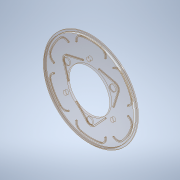
# Autodesk Inventor part: Top Lid
Saved by Autodesk Inventor 2020 (Build 240168000, 168)
## iProperties
Created: 2020-03-28
Part Number: Top Lid
Material: Generic
Document SubType Name: Modeling
Designer: pengpeng
Density: 1 g/cm^3
Appearance: Polycarbonate - Smoked
Author: pengpeng
Autodesk Inventor part; units mm, degrees
ref_plane "YZ Plane" through (0, 0, 0) normal (1, 0, 0) x (0, 1, 0)
ref_plane "XY Plane" through (0, 0, 0) normal (0, 0, 1) x (1, 0, 0)
sketch "Sketch1" plane through (0, 0, 0) normal (0, 0, 1) x (1, 0, 0)
  circle A0 centre (0, 0) radius 68
  dimension "d1" = 136
  constraints: 1 centre point
  measures "d1" diameter of A0
extrude "Extrusion1" add sketch "Sketch1" along normal blind 80
shell "Shell1" thickness 3 removed faces 1 at (13.6377, 7.7647, 0)
sketch "Sketch2" plane through (0, 0, 80) normal (0, 0, 1) x (1, 0, 0)
  circle A0 centre (0, 0) radius 32
  dimension "d5" = 64
  constraints: 1 centre point, 1 coincident
  measures "d5" diameter of A0
extrude "Extrusion2" cut sketch "Sketch2" against normal up to surface (3 mm away)
sketch "Sketch3" plane through (0, 0, 77) normal (0, 0, -1) x (-1, 0, 0)
  circle A0 centre (0, 0) radius 32 projected
  circle A1 centre (0, 0) radius 65 projected
  circle A2 centre (0, -40) radius 4.8
  line L0 (0, 0) -> (0, -56.282) construction
  line L1 (0, 0) -> (-47.9956, 27.7103) construction
  line L2 (0, 0) -> (60.1339, 34.7183) construction
  circle A3 centre (-34.641, 20) radius 4.8
  circle A4 centre (34.641, 20) radius 4.8
  dimension "d8" = 9.6
  dimension "d9" = 40
  dimension "d10" = 120
  dimension "d11" = 120
  dimension "d12" = 9.6
  dimension "d13" = 9.6
  dimension "d14" = 40
  dimension "d15" = 40
  constraints: 6 end point, 3 centre point, 2 point on line, 1 vertical
  measures "d8" diameter of A2
  measures "d9" distance of point (0, 0) A2.centre
  measures "d10" angle of L0 L1
  measures "d11" angle of L0 L2
  measures "d12" diameter of A3
  measures "d13" diameter of A4
  measures "d14" distance of point (0, 0) A4.centre
  measures "d15" distance of point (0, 0) A3.centre
extrude "Extrusion3" cut sketch "Sketch3" against normal blind 1.524 contours A2 | A3 | A4
ref_plane "Work Plane1" through (0, 0, 55) normal (0, 0, 1) x (1, 0, 0)
sketch "Sketch4" plane through (0, 0, 55) normal (0, 0, 1) x (1, 0, 0)
  circle A0 centre (0, 0) radius 68 projected
  circle A1 centre (0, 0) radius 68 projected
  line L0 (0, 68) -> (56.3915, 68)
  line L1 (56.3915, 68) -> (56.3915, 38)
  line L2 (56.3915, 38) -> (0, 38)
  line L3 (0, 38) -> (0, 68)
  dimension "d24" = 30
  constraints: 8 end point, 2 horizontal, 2 parallel, 1 perpendicular, 1 vertical alignment, 3 other
  measures "d24" distance between parallel lines of L2 L0
extrude "Extrusion4" add sketch "Sketch4" against normal blind 25 contours A0 L0 L1
sketch "Sketch6" plane through (56.3915, 38, 55) normal (1, 0, 0) x (0, 0, -1)
  line L0 (0, 0) -> (0, 30) projected
  line L1 (25, 0) -> (0, 0) projected
  line L2 (25, 30) -> (25, 0) projected
  line L3 (0, 30) -> (25, 30) projected
  line L4 (22, 27) -> (22, 3)
  line L5 (22, 3) -> (3, 3)
  line L6 (3, 3) -> (3, 27)
  line L7 (3, 27) -> (22, 27)
  point P0 (55, -38)
  dimension "d27" = 3
  constraints: 8 end point, 3 other
  measures "d27" distance between parallel lines of L3 L7
extrude "Extrusion5" cut sketch "Sketch6" against normal blind 56.391 contours L4 L5 L6 L7
ref_plane "Work Plane4" through (0, 68, 0) normal (0, 1, 0) x (-1, 0, 0)
sketch "Sketch9" plane through (56.3915, 38, 55) normal (1, 0, 0) x (0, 0, -1)
  line L0 (3, 3) -> (3, 27) projected
  line L1 (3, 27) -> (22, 27) projected
  line L2 (22, 27) -> (22, 3) projected
  line L3 (22, 3) -> (3, 3) projected
  line L4 (0, 0) -> (0, 30) projected
  line L5 (25, 0) -> (0, 0) projected
  line L6 (25, 30) -> (25, 0) projected
  line L7 (0, 30) -> (25, 30) projected
  point P0 (55, -38)
sketch "Sketch10" plane through (0, 68, 0) normal (0, 1, 0) x (-1, 0, 0)
  circle A0 centre (-56.3915, 0) radius 55 construction
  line L0 (-127.7058, 55) -> (100.6176, 55) projected
  line L1 (-56.3915, 55) -> (0, 55) projected
  line L2 (0, 0) -> (-96.3915, 0) construction
  arc A1 (-56.3915, 55) -> (-111.3915, 0) centre (-56.3915, 0) ccw
  constraints: 4 point on circle, 2 centre point, 2 coincident, 2 end point, 1 horizontal, 1 point on line, 1 tangent
sweep "Sweep2" add profiles "Sketch9" path "Sketch10" path curves A1
sketch "Sketch11" plane through (0, 0, 77) normal (0, 0, -1) x (-1, 0, 0)
  circle A0 centre (-34.641, 20) radius 4.8 projected
  circle A1 centre (34.641, 20) radius 4.8 projected
  circle A2 centre (0, -40) radius 4.8 projected
  circle A3 centre (0, 0) radius 32 projected
  circle A4 centre (0, 0) radius 65 projected
  circle A5 centre (-34.641, 20) radius 6.3
  circle A6 centre (34.641, 20) radius 6.3
  circle A7 centre (0, -40) radius 6.3
  circle A8 centre (0, 0) radius 33.5
  line L0 (-36.0415, 26.1424) -> (-7.4468, 32.6618)
  line L1 (-40.6607, 18.1416) -> (-32.0094, -9.8818)
  line L2 (36.0415, 26.1424) -> (7.4468, 32.6618)
  line L3 (40.6607, 18.1416) -> (32.0094, -9.8818)
  line L4 (4.6192, -44.284) -> (24.5626, -22.78)
  line L5 (-4.6192, -44.284) -> (-24.5626, -22.78)
  circle A9 centre (-34.641, 20) radius 7.8
  line L6 (-42.0939, 17.6992) -> (-34.7194, -6.1884)
  circle A10 centre (34.641, 20) radius 7.8
  circle A11 centre (0, -40) radius 7.8
  line L7 (-36.3749, 27.6048) -> (-12.0004, 33.1621)
  line L8 (36.3749, 27.6048) -> (12.0004, 33.1621)
  line L9 (42.0939, 17.6992) -> (34.7194, -6.1884)
  line L10 (5.7191, -45.304) -> (22.7191, -26.9737)
  line L11 (-5.7191, -45.304) -> (-22.7191, -26.9737)
  line L12 (-34.7194, -6.1884) -> (-33.2862, -5.746)
  line L13 (-22.7191, -26.9737) -> (-21.6192, -25.9537)
  line L14 (12.0004, 33.1621) -> (11.6669, 31.6997)
  line L15 (34.7194, -6.1884) -> (33.2862, -5.746)
  line L16 (22.7191, -26.9737) -> (21.6192, -25.9537)
  line L17 (-12.0004, 33.1621) -> (-11.6669, 31.6997)
  dimension "d39" = 1.5
  dimension "d40" = 1.5
  dimension "d41" = 1.5
  dimension "d42" = 1.5
  dimension "d43" = 1.5
  dimension "d44" = 1.5
  dimension "d45" = 1.5
  dimension "d46" = 25
  dimension "d47" = 25
  dimension "d48" = 25
  dimension "d49" = 25
  dimension "d50" = 25
  dimension "d51" = 25
  constraints: 36 end point, 18 point on circle, 18 tangent, 7 centre point, 6 parallel, 6 perpendicular, 6 point on line
  measures "d39" radial gap between concentric circles of A0 A5
  measures "d40" radial gap between concentric circles of A1 A6
  measures "d41" radial gap between concentric circles of A2 A7
  measures "d42" radial gap between concentric circles of A8 A3
  measures "d43" radial gap between concentric circles of A5 A9
  measures "d44" radial gap between concentric circles of A6 A10
  measures "d45" radial gap between concentric circles of A7 A11
  measures "d46" distance of L6.start L6.end
  measures "d47" distance of L7.start L7.end
  measures "d48" distance of L8.start L8.end
  measures "d49" distance of L9.start L9.end
  measures "d50" distance of L10.start L10.end
  measures "d51" distance of L11.start L11.end
extrude "Extrusion6" add sketch "Sketch11" along normal blind 1.5 contours A5 L1 A9 L0 | A9 L7 L17 L0 | L1 L12 L6 A9 | L14 L8 A10 L2 | L5 A11 L11 L13 | A10 L3 A6 L2 | L5 A7 L4 A11 | A10 L9 L15 L3 | L16 L10 A11 L4
sketch "Sketch14" plane through (0, 0, 80) normal (0, 0, 1) x (1, 0, 0)
  circle A0 centre (0, 0) radius 32 projected
  line L0 (0, 0) -> (0, 28.9416) construction
  circle A1 centre (0, 41) radius 3
  line L1 (0, 0) -> (-25.0642, -14.4708) construction
  line L2 (0, 0) -> (25.0642, -14.4708) construction
  point P0 (-35.507, -20.5)
  point P1 (-35.507, -20.5)
  point P2 (35.507, -20.5)
  point P3 (35.507, -20.5)
  dimension "d98" = 6
  dimension "d99" = 41
  dimension "d102" = 360
  constraints: 6 end point, 3 coincident, 3 point on line, 1 centre point, 1 vertical, 16 other
  measures "d98" diameter of A1
  measures "d99" distance of point (0, 0) A1.centre
hole "Hole1" at (0, 41, 80) at (-35.507, -20.5, 80) at (35.507, -20.5, 80) direction (0, 0, -1) diameter 6 end through all
sketch "Sketch16" plane through (0, 0, 0) normal (0, 0, -1) x (-1, 0, 0)
  circle A0 centre (0, 0) radius 68 projected
  line L0 (-147.0847, -150.1925) -> (110.1745, -150.1925)
  line L1 (110.1745, -150.1925) -> (110.1745, 168.3901)
  line L2 (110.1745, 168.3901) -> (-147.0847, 168.3901)
  line L3 (-147.0847, 168.3901) -> (-147.0847, -150.1925)
  constraints: 8 end point, 2 parallel, 1 horizontal, 1 perpendicular
extrude "Extrusion9" cut sketch "Sketch16" against normal up to surface (75.5 mm away) contours A0 | L3 L2 L1 L0
sketch "Sketch17" plane through (0, 0, 75.5) normal (0, 0, -1) x (-1, 0, 0)
  circle A0 centre (0, 0) radius 65 projected
  circle A1 centre (0, 0) radius 68 projected
extrude "Extrusion10" cut sketch "Sketch17" against normal up to surface (1.5 mm away)
sketch "Sketch18" plane through (0, 0, 77) normal (0, 0, -1) x (-1, 0, 0)
  circle A0 centre (0, 0) radius 68 projected
  circle A1 centre (0, 0) radius 71
  line L0 (0, 0) -> (-80.0299, 0) construction
  circle A2 centre (-57.5, 0) radius 4.8
  circle A3 centre (0, 0) radius 65
  circle A4 centre (-57.5, 0) radius 6.3
  circle A5 centre (-52.744, -15.5907) radius 10
  circle A6 centre (-52.744, 15.5907) radius 10
  circle A7 centre (-12.87, -53.473) radius 10
  circle A8 centre (-28.75, -49.7965) radius 6.3
  circle A9 centre (-28.75, -49.7965) radius 4.8
  circle A10 centre (-39.874, -37.8823) radius 10
  circle A11 centre (39.874, -37.8823) radius 10
  circle A12 centre (28.75, -49.7965) radius 6.3
  circle A13 centre (28.75, -49.7965) radius 4.8
  circle A14 centre (12.87, -53.473) radius 10
  circle A15 centre (52.744, 15.5907) radius 10
  circle A16 centre (57.5, 0) radius 6.3
  circle A17 centre (57.5, 0) radius 4.8
  circle A18 centre (52.744, -15.5907) radius 10
  circle A19 centre (12.87, 53.473) radius 10
  circle A20 centre (28.75, 49.7965) radius 6.3
  circle A21 centre (28.75, 49.7965) radius 4.8
  circle A22 centre (39.874, 37.8823) radius 10
  circle A23 centre (-39.874, 37.8823) radius 10
  circle A24 centre (-28.75, 49.7965) radius 6.3
  circle A25 centre (-28.75, 49.7965) radius 4.8
  circle A26 centre (-12.87, 53.473) radius 10
  circle A27 centre (-52.744, -15.5907) radius 8.5
  circle A28 centre (-39.874, -37.8823) radius 8.5
  circle A29 centre (0, 0) radius 63.5
  line L1 (-33.0494, -45.1916) -> (-34.0731, -44.0952)
  line L2 (-55.6618, -6.0259) -> (-55.2241, -7.4606)
  circle A30 centre (-12.87, -53.473) radius 8.5
  circle A31 centre (12.87, -53.473) radius 8.5
  line L3 (-22.6123, -51.2175) -> (-21.151, -51.5558)
  line L4 (22.6123, -51.2175) -> (21.151, -51.5558)
  circle A32 centre (39.874, -37.8823) radius 8.5
  circle A33 centre (52.744, -15.5907) radius 8.5
  line L5 (33.0494, -45.1916) -> (34.0731, -44.0952)
  line L6 (55.6618, -6.0259) -> (55.2241, -7.4606)
  circle A34 centre (52.744, 15.5907) radius 8.5
  circle A35 centre (39.874, 37.8823) radius 8.5
  line L7 (55.6618, 6.0259) -> (55.2241, 7.4606)
  line L8 (33.0494, 45.1916) -> (34.0731, 44.0952)
  circle A36 centre (12.87, 53.473) radius 8.5
  circle A37 centre (-12.87, 53.473) radius 8.5
  line L9 (22.6123, 51.2175) -> (21.151, 51.5558)
  line L10 (-22.6123, 51.2175) -> (-21.151, 51.5558)
  circle A38 centre (-39.874, 37.8823) radius 8.5
  circle A39 centre (-52.744, 15.5907) radius 8.5
  line L11 (-33.0494, 45.1916) -> (-34.0731, 44.0952)
  line L12 (-55.6618, 6.0259) -> (-55.2241, 7.4606)
  point P0 (22.6123, -51.2175)
  point P1 (14.859, -61.737)
  point P2 (-14.859, -61.737)
  point P3 (-22.6123, -51.2175)
  point P4 (-15.2101, -63.1954)
  point P5 (15.2101, -63.1954)
  point P6 (55.6618, -6.0259)
  point P7 (60.8953, -18.0002)
  point P8 (46.0363, -43.7368)
  point P9 (33.0494, -45.1916)
  point P10 (47.1238, -44.77)
  point P11 (62.3338, -18.4254)
  point P12 (33.0494, 45.1916)
  point P13 (46.0363, 43.7368)
  point P14 (60.8953, 18.0002)
  point P15 (55.6618, 6.0259)
  point P16 (62.3338, 18.4254)
  point P17 (47.1238, 44.77)
  point P18 (-22.6123, 51.2175)
  point P19 (-14.859, 61.737)
  point P20 (14.859, 61.737)
  point P21 (15.2101, 63.1954)
  point P22 (-15.2101, 63.1954)
  point P23 (-55.6618, 6.0259)
  point P24 (-60.8953, 18.0002)
  point P25 (-46.0363, 43.7368)
  point P26 (-33.0494, 45.1916)
  point P27 (-47.1238, 44.77)
  point P28 (-62.3338, 18.4254)
  point P29 (-60.8953, -18.0002)
  point P30 (-62.3338, -18.4254)
  point P31 (-47.1238, -44.77)
  point P32 (-46.0363, -43.7368)
  dimension "d120" = 20
  dimension "d126" = 1.5
  dimension "d127" = 1.5
  dimension "d115" = 142
  dimension "d116" = 9.6
  dimension "d117" = 130
  dimension "d118" = 57.5
  dimension "d119" = 1.5
  dimension "d121" = 20
  dimension "d124" = 360
  dimension "d130" = 360
  constraints: 26 end point, 23 centre point, 2 coincident, 1 horizontal, 1 point on line, 1 tangent, 157 other
  measures "d115" diameter of A1
  measures "d116" diameter of A2
  measures "d117" diameter of A3
  measures "d118" distance of point (0, 0) A2.centre
  measures "d121" diameter of A6
extrude "Extrusion11" add sketch "Sketch18" along normal blind 1.5 contours A1 | A15 A29 A22 A3 | A15 A29 | A3 A11 A29 A18 | A18 A29 | A22 A29 | A11 A29 | A19 A29 A26 A3 | A19 A29 | A29 A35 L8 A22 | A15 L7 A34 A29 | A3 A7 A29 A14 | A14 A29 | A11 L5 A32 A29 | A18 A29 A33 L6 | A26 A29 | A19 L9 A36 A29 | A7 A29 | A29 A31 L4 A14 | A23 A29 A6 A3 | A23 A29 | A29 A37 L10 A26 | A3 A5 A29 A10 | A10 A29 | A7 L3 A30 A29 | A6 A29 | A23 L11 A38 A29 | A5 A29 | A29 A28 L1 A10 | A29 A39 L12 A6 | A5 L2 A27 A29 picked at (34.5421, 45.674) picked at (56.7995, 7.0624) picked at (34.5421, -45.6741) picked at (56.7995, -7.0624) picked at (22.201, 54.9051) picked at (22.201, -54.9051) picked at (-22.2838, 52.7514) picked at (-22.2838, -52.7514) picked at (-34.5421, 45.6741) picked at (-34.5421, -45.674) picked at (-56.826, 7.0773) picked at (-56.826, -7.0773)
equation "\"d11\" = d10"
equation "\"d12\" = d8"
equation "\"d13\" = d8"
equation "\"d14\" = d9"
equation "\"d15\" = d9"
equation "\"d40\" = d39"
equation "\"d41\" = d39"
equation "\"d42\" = d39"
equation "\"d44\" = d43"
equation "\"d45\" = d41"
equation "\"d47\" = d46"
equation "\"d48\" = d47"
equation "\"d49\" = d48"
equation "\"d50\" = d49"
equation "\"d51\" = d50"
equation "\"d127\" = d126"
equation "\"d121\" = d120"
body "Solid1"
